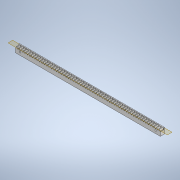
# Autodesk Inventor part: Rack
Saved by Autodesk Inventor 2022 (Build 260153000, 153)
## iProperties
Created: 2022-08-19
Part Number: Rack
Material: Generico
Document SubType Name: Modeling
Designer: matte
Density: 1 g/cm^3
Appearance: Default
Author: matte
Autodesk Inventor part; units mm, degrees
ref_plane "YZ Plane" through (0, 0, 0) normal (1, 0, 0) x (0, 1, 0)
ref_plane "XZ Plane" through (0, 0, 0) normal (0, 1, 0) x (-1, 0, 0)
ref_plane "XY Plane" through (0, 0, 0) normal (0, 0, 1) x (1, 0, 0)
sketch "Rettangolo base" plane through (0, 0, 0) normal (0, 0, 1) x (1, 0, 0)
  line L0 (-188.4956, 5.25) -> (188.4956, 5.25)
  line L1 (188.4956, 5.25) -> (188.4956, -5.25)
  line L2 (188.4956, -5.25) -> (-188.4956, -5.25)
  line L3 (-188.4956, -5.25) -> (-188.4956, 5.25)
  point P0 (0, 0)
  point P1 (0, 5.25)
  point P2 (188.4956, 0)
  dimension "d0" = 376.9911
  dimension "d1" = 10.5
  constraints: 8 end point, 2 midpoint, 2 parallel, 1 horizontal, 1 horizontal alignment, 1 perpendicular, 1 vertical alignment
  measures "d0" distance of L1.end L2.end
  measures "d1" distance between parallel lines of L0 L2
extrude "Estrusione1" add sketch "Rettangolo base" along normal blind 11
sketch "Trapezio dente" plane through (0, 0, 11) normal (0, 0, 1) x (1, 0, 0)
  line L0 (-187.8347, 5.25) -> (-186.1968, 9.75)
  line L1 (-186.1968, 9.75) -> (-184.5111, 9.75)
  line L2 (-184.5111, 9.75) -> (-182.8732, 5.25)
  line L3 (-185.354, 38.945) -> (-185.354, 10.1058) construction
  line L4 (188.4956, 5.25) -> (-188.4956, 5.25) construction
  line L5 (-186.9248, 7.75) -> (-183.7832, 7.75) construction
  line L6 (-187.8347, 5.25) -> (-182.8732, 5.25)
  line L7 (-188.4956, 5.25) -> (-188.4956, -5.25) projected
  point P0 (0, 0)
  dimension "d4" = 40
  dimension "d6" = 2
  dimension "d7" = 3.1416
  dimension "d15" = 3.1416
  dimension "d25" = 2.5
  constraints: 12 end point, 4 point on line, 2 horizontal, 1 parallel, 1 vertical, 1 other
  measures "d4" angle of L2 L0
  measures "d6" distance between parallel lines of L1 L5
  measures "d7" distance of L5.start L5.end
  measures "d15" distance between parallel lines of L7 L3
  measures "d25" distance between parallel lines of L5 L4
extrude "Estrusione2" add sketch "Trapezio dente" against normal blind 9
fillet "Raccordo1" radius 0.9 1 edges at (-182.8732, 5.25, 6.5)
fillet "Raccordo1" radius 0.9 1 edges at (-187.8347, 5.25, 6.5)
pattern_linear "Serie rettangolare1" count 60 spacing 6.2832 along (1, 0, 0) of "Estrusione2", "Raccordo1"
sketch "Schizzo fori" plane through (0, 0, 11) normal (0, 0, 1) x (1, 0, 0)
  line L0 (-188.4956, 5.25) -> (-188.4956, -5.25) projected
  line L1 (188.4956, -5.25) -> (188.4956, 5.25) projected
  line L2 (-188.4956, -5.25) -> (188.4956, -5.25) projected
  point P0 (0, 0)
  point P1 (-176.4956, 2.25)
  point P2 (176.4956, 2.25)
  dimension "d16" = 12
  dimension "d17" = 12
  dimension "d34" = 7.5
  dimension "d35" = 7.5
  measures "d16" distance from line of L0 point (-176.496, 2.25)
  measures "d17" distance from line of L1 point (176.496, 2.25)
  measures "d34" distance from line of L2 point (-176.496, 2.25)
  measures "d35" distance from line of L2 point (176.496, 2.25)
hole "Foro1" at (-176.4956, 2.25, 11) at (176.4956, 2.25, 11) direction (0, 0, -1) diameter 4 end through all
sketch "Schizzo5" plane through (-188.4956, 5.25, 0) normal (0, 1, 0) x (1, 0, 0)
  line L0 (376.9911, 0) -> (0, 0) projected
  line L1 (376.9911, 0) -> (376.9911, -11) projected
  line L2 (365.3012, -2) -> (366.7235, -2) projected
  line L3 (0, 0) -> (0, -11) projected
  line L4 (376.9911, -2) -> (0, -2)
  line L5 (0, -2) -> (0, 0)
  line L6 (0, 0) -> (376.9911, 0)
  line L7 (376.9911, 0) -> (376.9911, -2)
  line L8 (366.7235, -2) -> (368.4092, -2) projected
  point P0 (188.4956, 0)
  point P1 (0, -2)
  point P2 (365.0856, 1)
  dimension "d26" = 0
  dimension "d27" = 0
  dimension "d28" = 0
  dimension "d29" = 0
  constraints: 6 end point, 1 horizontal, 1 parallel, 1 vertical, 4 other
  measures "d26" distance between parallel lines of L7 L1
  measures "d27" distance between parallel lines of L0 L6
  measures "d28" vertical extent of L8
  measures "d29" distance between parallel lines of L3 L5
extrude "Estrusione3" add sketch "Schizzo5" along normal blind 4.5
ref_plane "Piano di lavoro1" through (-188.4956, 7.75, 0) normal (0, 1, 0) x (1, 0, 0)
equation "\"d2\" = spessore_body"
equation "\"d7\" = 1.5708 * m_val"
equation "\"d15\" = 1.5708 * m_val"
equation "\"d8\" = spessore_dente"
equation "\"d14\" = 3.14159 * m_val"
equation "\"d17\" = d16"
equation "\"spessore_dente\" = 9"
equation "\"spessore_body\" = 11"
equation "\"m_val\" = 2"
equation "\"r_racc\" = 0.9"
equation "\"base\" = 15"
